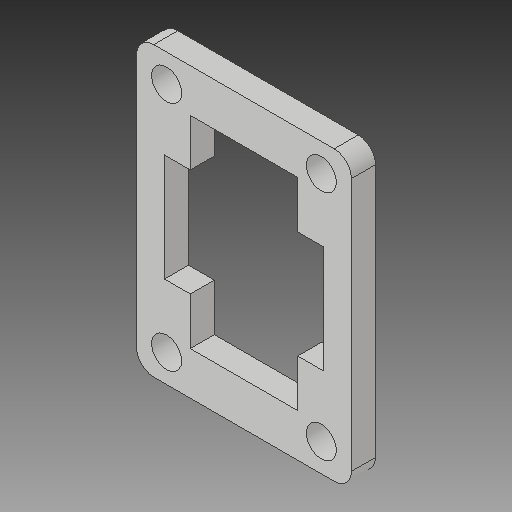
# Autodesk Inventor part: Part20
Saved by Autodesk Inventor 2019.2 (Build 232265000, 265)
## iProperties
Created: 2019-04-01
Part Number: Part20
Material: Generic
Document SubType Name: Modeling
Designer: richard.girt
Mass: 1.19513 g
Surface Area: 15.3 cm^2
Volume: 1.19513 cm^3
Density: 1 g/cm^3
Appearance: Default
Author: richard.girt
Autodesk Inventor part; units mm, degrees
ref_plane "YZ Plane" through (0, 0, 0) normal (1, 0, 0) x (0, 1, 0)
ref_plane "XZ Plane" through (0, 0, 0) normal (0, 1, 0) x (-1, 0, 0)
ref_plane "XY Plane" through (0, 0, 0) normal (0, 0, 1) x (1, 0, 0)
sketch "Sketch1" plane through (0, 0, 0) normal (0, 0, 1) x (1, 0, 0)
  line L0 (6.25, -11.75) -> (-6.25, -11.75)
  line L1 (-6.25, -11.75) -> (-6.25, 11.75)
  line L2 (-6.25, 11.75) -> (6.25, 11.75)
  line L3 (6.25, 11.75) -> (6.25, -11.75)
  line L4 (6.25, -11.75) -> (-6.25, 11.75) construction
  line L5 (-6.25, -11.75) -> (6.25, 11.75) construction
  line L6 (9.25, 6.25) -> (-9.25, 6.25)
  line L7 (-9.25, 6.25) -> (-9.25, -6.25)
  line L8 (-9.25, -6.25) -> (9.25, -6.25)
  line L9 (9.25, -6.25) -> (9.25, 6.25)
  line L10 (9.25, 6.25) -> (-9.25, -6.25) construction
  line L11 (-9.25, 6.25) -> (9.25, -6.25) construction
  line L12 (-10.5, 16.75) -> (10.5, 16.75)
  line L13 (12.5, 14.75) -> (12.5, -14.75)
  line L14 (10.5, -16.75) -> (-10.5, -16.75)
  line L15 (-12.5, -14.75) -> (-12.5, 14.75)
  line L16 (-9, -13.5) -> (9, -13.5) construction
  circle A0 centre (-9, -13.5) radius 1.75
  circle A1 centre (9, -13.5) radius 1.75
  circle A2 centre (-9, 13.5) radius 1.75
  circle A3 centre (9, 13.5) radius 1.75
  arc A4 (-10.5, 16.75) -> (-12.5, 14.75) centre (-10.5, 14.75) ccw
  arc A5 (12.5, 14.75) -> (10.5, 16.75) centre (10.5, 14.75) ccw
  arc A6 (10.5, -16.75) -> (12.5, -14.75) centre (10.5, -14.75) ccw
  arc A7 (-12.5, -14.75) -> (-10.5, -16.75) centre (-10.5, -14.75) ccw
  point P0 (0, 0)
  point P1 (-12.5, 16.75)
  point P2 (12.5, 16.75)
  point P3 (-12.5, -16.75)
  point P4 (0, 16.75)
  point P5 (0, 0)
  point P6 (0, -23.5)
  point P7 (0, 0)
  dimension "d0" = 33.5
  dimension "d1" = 25
  dimension "d2" = 23.5
  dimension "d3" = 12.5
  dimension "d4" = 18.5
  dimension "d5" = 12.5
  dimension "d6" = 16.75
  dimension "d12" = 2
  dimension "d16" = 9
  dimension "d17" = 18
  dimension "d18" = 13.5
  dimension "d19" = 27
  dimension "d20" = 3.5
  constraints: 34 end point, 8 centre point, 8 point on circle, 8 tangent, 7 midpoint, 6 equal radius, 6 parallel, 6 point on line, 4 horizontal, 4 vertical alignment, 3 perpendicular, 2 coincident, 1 horizontal alignment
  measures "d0" distance of point (-12.5, -16.75) point (-12.5, 16.75)
  measures "d1" distance of point (-12.5, 16.75) point (12.5, 16.75)
  measures "d2" distance of L0.end L1.end
  measures "d3" distance of L1.end L2.end
  measures "d4" distance of L7.end L8.end
  measures "d5" distance of L8.end L6.start
  measures "d6" distance from line of L12 point (0, 0)
  measures "d12" radius of A4
  measures "d16" horizontal distance of A2.centre point (0, 16.75)
  measures "d17" distance of A3.centre A2.centre
  measures "d18" vertical distance of A3.centre point (0, 0)
  measures "d19" distance of L16.end A3.centre
  measures "d20" diameter of A1
extrude "Extrusion1" add sketch "Sketch1" against normal blind 2.8
equation "\"d0\" = 2 * d6"
body "Solid1"
